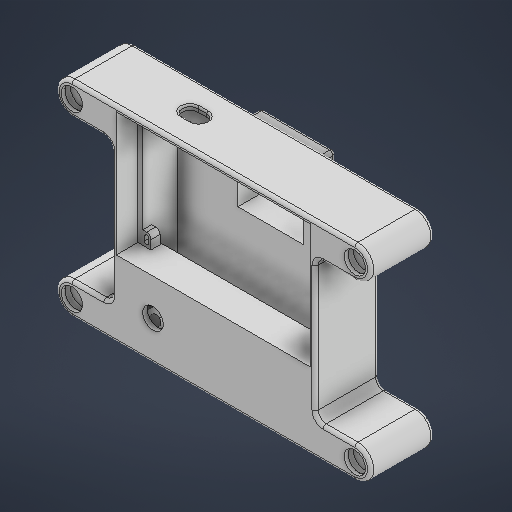
# Autodesk Inventor part: door-opener-v2-enclosure
Saved by Autodesk Inventor 2026.2 (Build 302298010, 298A)
## iProperties
Created: 2025-11-21
Part Number: door-opener-v2-enclosure
Material: Generic
Document SubType Name: Modeling
Designer: ericswpark
Density: 1 g/cm^3
Appearance: Default
Author: ericswpark
Autodesk Inventor part; units mm, degrees
ref_plane "YZ Plane" through (0, 0, 0) normal (1, 0, 0) x (0, 1, 0)
ref_plane "XZ Plane" through (0, 0, 0) normal (0, 1, 0) x (-1, 0, 0)
ref_plane "XY Plane" through (0, 0, 0) normal (0, 0, 1) x (1, 0, 0)
sketch "Sketch1" plane through (0, 0, 0) normal (0, 0, 1) x (1, 0, 0)
  line L0 (0, 0) -> (128.3, 0)
  line L1 (128.3, 0) -> (128.3, 129.1)
  line L2 (128.3, 129.1) -> (0, 129.1)
  line L3 (0, 129.1) -> (0, 0)
  circle A0 centre (153.3, 119.1) radius 10
  line L4 (128.3, 129.1) -> (153.3, 129.1)
  line L5 (153.3, 129.1) -> (153.3, 109.1)
  line L6 (153.3, 109.1) -> (128.3, 109.1)
  line L7 (128.3, 109.1) -> (128.3, 129.1)
  circle A1 centre (153.3, 119.1) radius 7
  circle A2 centre (-25, 119.1) radius 7
  circle A3 centre (-25, 119.1) radius 10
  line L8 (-25, 109.1) -> (0, 109.1)
  line L9 (0, 109.1) -> (0, 129.1)
  line L10 (0, 129.1) -> (-25, 129.1)
  line L11 (-25, 129.1) -> (-25, 109.1)
  circle A4 centre (153.3, 10) radius 7
  circle A5 centre (153.3, 10) radius 10
  line L12 (153.3, 20) -> (128.3, 20)
  line L13 (128.3, 20) -> (128.3, 0)
  line L14 (128.3, 0) -> (153.3, 0)
  line L15 (153.3, 0) -> (153.3, 20)
  line L16 (0, 20) -> (-25, 20)
  line L17 (-25, 20) -> (-25, 0)
  line L18 (-25, 0) -> (0, 0)
  line L19 (0, 0) -> (0, 20)
  circle A6 centre (-25, 10) radius 7
  circle A7 centre (-25, 10) radius 10
  point P0 (153.3, 0)
  point P1 (0, 20)
  point P2 (-25, 129.1)
  point P3 (-25, 109.1)
  point P4 (0, 109.1)
  point P5 (128.3, 109.1)
  point P6 (153.3, 109.1)
  point P7 (153.3, 129.1)
  dimension "d0" = 128.3
  dimension "d1" = 129.1
  dimension "d87" = 25
  dimension "d88" = 20
  dimension "d89" = 14
  dimension "d90" = 14
  dimension "d91" = 20
  dimension "d92" = 25
  dimension "d93" = 14
  dimension "d94" = 20
  dimension "d95" = 25
  dimension "d96" = 14
  dimension "d97" = 20
  dimension "d98" = 25
  constraints: 40 end point, 10 parallel, 8 centre point, 8 tangent, 6 midpoint, 5 horizontal, 5 perpendicular, 4 coincident, 3 point on line
  measures "d0" distance between parallel lines of L1 L3
  measures "d1" distance between parallel lines of L0 L2
  measures "d87" distance from line of L1 point (153.3, 119.1)
  measures "d88" diameter of A0
  measures "d89" diameter of A1
  measures "d90" diameter of A2
  measures "d91" diameter of A3
  measures "d92" distance from line of L3 point (-25, 119.1)
  measures "d93" diameter of A6
  measures "d94" diameter of A7
  measures "d95" distance from line of L3 A6.centre
  measures "d96" diameter of A4
  measures "d97" diameter of A5
  measures "d98" distance from line of L1 A4.centre
extrude "Initial extrusion" add sketch "Sketch1" along normal blind 40
sketch "Sketch2" plane through (0, 0, 0) normal (0, 0, -1) x (-1, 0, 0)
  line L0 (-6, 0) -> (-122.3, 0)
  line L1 (-122.3, 0) -> (-122.3, 123.1)
  line L2 (-122.3, 123.1) -> (-6, 123.1)
  line L3 (-6, 123.1) -> (-6, 0)
  line L4 (0, 109.1) -> (0, 0) projected
  line L5 (-128.3, 20) -> (-128.3, 109.1) projected
  line L6 (-153.3, 129.1) -> (25, 129.1) projected
  line L7 (25, 0) -> (-153.3, 0) projected
  dimension "d4" = 6
  dimension "d5" = 6
  dimension "d180" = 6
  constraints: 8 end point, 2 parallel, 1 collinear, 1 horizontal, 1 perpendicular
  measures "d4" distance between parallel lines of L4 L3
  measures "d5" distance between parallel lines of L1 L5
  measures "d180" distance between parallel lines of L2 L6
extrude "Top cutout" cut sketch "Sketch2" against normal blind 3
sketch "Sketch3" plane through (0, 0, 40) normal (0, -1, 0) x (1, 0, 0)
  line L0 (125.3, -37) -> (3, -37)
  line L1 (3, -37) -> (3, -35.5)
  line L2 (3, -35.5) -> (125.3, -35.5)
  line L3 (125.3, -35.5) -> (125.3, -37)
  line L4 (6, -37) -> (122.3, -37) projected
  line L5 (122.3, -37) -> (122.3, -40) projected
  line L6 (6, -40) -> (6, -37) projected
  dimension "d11" = 1.5
  dimension "d181" = 3
  dimension "d182" = 3
  constraints: 8 end point, 2 parallel, 1 collinear, 1 horizontal, 1 perpendicular
  measures "d11" distance between parallel lines of L0 L2
  measures "d181" distance between parallel lines of L5 L3
  measures "d182" distance between parallel lines of L1 L6
extrude "BP slide section" cut sketch "Sketch3" against normal blind 126.6
sketch "Sketch4" plane through (125.3, 0, 4.5) normal (0, 0, -1) x (-1, 0, 0)
  line L0 (119.3, 3) -> (3, 3)
  line L1 (3, 3) -> (3, 126.1)
  line L2 (3, 126.1) -> (119.3, 126.1)
  line L3 (119.3, 126.1) -> (119.3, 3)
  line L4 (0, 0) -> (0, 126.6) projected
  line L5 (122.3, 0) -> (122.3, 126.6) projected
  line L6 (122.3, 0) -> (0, 0) projected
  line L7 (-28, 129.1) -> (150.3, 129.1) projected
  point P0 (125.3, 0)
  point P1 (0, 123.1)
  dimension "d15" = 3
  dimension "d16" = 3
  dimension "d183" = 3
  dimension "d184" = 3
  constraints: 8 end point, 2 parallel, 1 horizontal, 1 perpendicular
  measures "d15" distance between parallel lines of L1 L4
  measures "d16" distance between parallel lines of L5 L3
  measures "d183" distance between parallel lines of L6 L0
  measures "d184" distance between parallel lines of L2 L7
extrude "Inner cavity" cut sketch "Sketch4" against normal blind 32.5
sketch "Sketch6" plane through (125.3, 0, 37) normal (0, 0, -1) x (-1, 0, 0)
  circle A0 centre (5.5, 121) radius 2.75
  circle A1 centre (116.8, 121) radius 2.75
  arc A2 (3, 54.7456) -> (3, 52.4544) centre (5.5, 53.6) ccw construction
  line L0 (3, 126.1) -> (119.3, 126.1) projected
  line L1 (3, 3) -> (3, 126.1) projected
  line L2 (119.3, 126.1) -> (119.3, 3) projected
  line L3 (3, 0) -> (3, 126.1) projected
  line L4 (3, 50.85) -> (3, 56.35)
  line L5 (3, 56.35) -> (5.5, 56.35)
  line L6 (5.5, 56.35) -> (5.5, 50.85) construction
  line L7 (3, 126.1) -> (8.25, 126.1)
  line L8 (8.25, 126.1) -> (8.25, 118.25)
  line L9 (8.25, 118.25) -> (3, 118.25)
  line L10 (3, 118.25) -> (3, 126.1)
  line L11 (119.3, 126.1) -> (114.05, 126.1)
  line L12 (114.05, 126.1) -> (114.05, 118.25)
  line L13 (114.05, 118.25) -> (119.3, 118.25)
  line L14 (119.3, 118.25) -> (119.3, 126.1)
  arc A3 (6.85, 53.6) -> (4.15, 53.6) centre (5.5, 53.6) ccw
  circle A4 centre (116.8, 121) radius 1.35
  circle A5 centre (5.5, 121) radius 1.35
  line L15 (3, 56.35) -> (8.25, 56.35) construction
  line L16 (8.25, 56.35) -> (8.25, 53.6) construction
  line L17 (8.25, 48) -> (3, 48)
  line L18 (3, 48) -> (3, 56.35)
  line L19 (8.25, 53.6) -> (8.25, 48)
  arc A6 (5.5, 56.35) -> (3, 54.7456) centre (5.5, 53.6) ccw construction
  arc A7 (3, 52.4544) -> (8.25, 53.6) centre (5.5, 53.6) ccw construction
  arc A8 (8.25, 53.6) -> (5.5, 56.35) centre (5.5, 53.6) ccw
  line L20 (4.15, 53.6) -> (6.85, 53.6) construction
  line L21 (6.85, 53.6) -> (6.85, 50.85)
  line L22 (5.5, 50.85) -> (4.15, 50.85) construction
  line L23 (4.15, 50.85) -> (4.15, 53.6)
  line L24 (4.15, 50.85) -> (3, 50.85) construction
  arc A9 (4.15, 50.85) -> (6.85, 50.85) centre (5.5, 50.85) ccw
  line L25 (116.8, 121) -> (5.5, 121) construction
  line L26 (61.15, 121) -> (61.15, 42.4019) construction
  arc A10 (119.3, 52.4544) -> (119.3, 54.7456) centre (116.8, 53.6) ccw construction
  line L27 (119.3, 3) -> (119.3, 126.1)
  line L28 (119.3, 50.85) -> (119.3, 56.35)
  line L29 (119.3, 56.35) -> (116.8, 56.35)
  line L30 (116.8, 56.35) -> (116.8, 50.85) construction
  arc A11 (118.15, 53.6) -> (115.45, 53.6) centre (116.8, 53.6) ccw
  line L31 (119.3, 56.35) -> (114.05, 56.35) construction
  line L32 (114.05, 56.35) -> (114.05, 53.6) construction
  line L33 (114.05, 48) -> (119.3, 48)
  line L34 (119.3, 48) -> (119.3, 56.35)
  line L35 (114.05, 53.6) -> (114.05, 48)
  arc A12 (119.3, 54.7456) -> (116.8, 56.35) centre (116.8, 53.6) ccw construction
  arc A13 (114.05, 53.6) -> (119.3, 52.4544) centre (116.8, 53.6) ccw construction
  arc A14 (116.8, 56.35) -> (114.05, 53.6) centre (116.8, 53.6) ccw
  line L36 (118.15, 53.6) -> (115.45, 53.6) construction
  line L37 (115.45, 53.6) -> (115.45, 50.85)
  line L38 (116.8, 50.85) -> (118.15, 50.85) construction
  line L39 (118.15, 50.85) -> (118.15, 53.6)
  line L40 (118.15, 50.85) -> (119.3, 50.85) construction
  arc A15 (115.45, 50.85) -> (118.15, 50.85) centre (116.8, 50.85) ccw
  point P0 (125.3, 0)
  point P1 (1, 0)
  point P2 (5.5, 56.35)
  point P3 (3, 56.35)
  point P4 (114.05, 121)
  point P5 (116.8, 118.25)
  point P6 (5.5, 118.25)
  point P7 (8.25, 121)
  point P8 (3, 118.25)
  point P9 (3, 48)
  dimension "d26" = 5.1
  dimension "d27" = 2.5
  dimension "d28" = 5.1
  dimension "d29" = 2.5
  dimension "d34" = 5.5
  dimension "d35" = 5.5
  dimension "d46" = 2.7
  dimension "d48" = 2.7
  dimension "d49" = 2.7
  dimension "d178" = 2.5
  dimension "d179" = 5.5
  dimension "d190" = 67.4
  dimension "d211" = 2.85
  dimension "d212" = 78.5981
  constraints: 74 end point, 26 point on circle, 18 symmetric about line, 18 tangent, 16 centre point, 11 parallel, 6 coincident, 6 midpoint, 6 perpendicular, 5 horizontal, 2 point on line, 1 collinear, 1 vertical, 8 other
  measures "d26" distance from line of L0 A0.centre
  measures "d27" distance from line of L1 A0.centre
  measures "d28" distance from line of L0 A1.centre
  measures "d29" distance from line of L2 A1.centre
  measures "d34" diameter of A0
  measures "d35" diameter of A1
  measures "d46" diameter of A3
  measures "d48" diameter of A4
  measures "d49" diameter of A5
  measures "d178" distance from line of L1 A3.centre
  measures "d179" diameter of A2
  measures "d190" distance of point (5.5, 53.6) A0.centre
  measures "d211" distance between parallel lines of L17 L24
  measures "d212" distance of L26.start L26.end
extrude "Display mount holes" add sketch "Sketch6" along normal blind 16.3 contours A0 L1 | A0 L1 L0 L8 | L9 L1 A0 | L2 A1 | A1 L12 L0 L2 | L2 L13 A1 | L1 L5 A8 L19 L17 | L2 L33 L35 A14 L29 picked at (3.3833, 121) picked at (118.9167, 121)
sketch "Sketch7" plane through (0, 0, 40) normal (0, 0, 1) x (1, 0, 0)
  line L0 (3, 126.1) -> (125.3, 126.1)
  line L1 (125.3, 126.1) -> (125.3, 48)
  line L2 (125.3, 48) -> (3, 48)
  line L3 (3, 48) -> (3, 126.1)
  line L4 (0, 109.1) -> (0, 0) projected
  line L5 (128.3, 20) -> (128.3, 109.1) projected
  line L6 (153.3, 129.1) -> (-25, 129.1) projected
  point P0 (124.3, 0)
  dimension "d40" = 3
  dimension "d42" = 3
  dimension "d43" = 78.1
  dimension "d185" = 3
  constraints: 8 end point, 2 parallel, 1 horizontal, 1 perpendicular, 1 other
  measures "d40" distance between parallel lines of L4 L3
  measures "d43" distance between parallel lines of L0 L2
  measures "d185" distance between parallel lines of L0 L6
extrude "Display cutout" cut sketch "Sketch7" against normal blind 13.6
sketch "Sketch9" plane through (125.3, 0, 37) normal (0, 0, -1) x (-1, 0, 0)
  line L0 (3, 3) -> (3, 48) projected
  line L1 (119.3, 48) -> (119.3, 3) projected
  line L2 (3, 48) -> (119.3, 48)
  line L3 (119.3, 48) -> (119.3, 46)
  line L4 (119.3, 46) -> (3, 46)
  line L5 (3, 46) -> (3, 48)
  point P0 (125.3, 0)
  point P1 (119.3, 48)
  point P2 (3, 46)
  dimension "d50" = 2
  constraints: 8 end point, 2 parallel, 1 horizontal, 1 perpendicular, 1 point on line
  measures "d50" distance between parallel lines of L2 L4
extrude "Separator" add sketch "Sketch9" along normal blind 17.5
sketch "Sketch10" plane through (125.3, 0, 37) normal (0, 0, -1) x (-1, 0, 0)
  circle A0 centre (11, 38) radius 2.25
  circle A1 centre (39, 12) radius 2.25
  circle A2 centre (39, 12) radius 3.25
  circle A3 centre (11, 38) radius 3.25
  line L0 (119.3, 46) -> (3, 46) projected
  line L1 (3, 3) -> (3, 46) projected
  point P0 (125.3, 0)
  dimension "d53" = 4.5
  dimension "d54" = 6.5
  dimension "d55" = 8
  dimension "d56" = 8
  dimension "d57" = 4.5
  dimension "d58" = 6.5
  dimension "d59" = 28
  dimension "d60" = 26
  constraints: 4 centre point, 2 coincident
  measures "d53" diameter of A0
  measures "d54" diameter of A3
  measures "d55" distance from line of A0.centre L0
  measures "d56" distance from line of L1 A0.centre
  measures "d57" diameter of A1
  measures "d58" diameter of A2
  measures "d59" horizontal distance of A0.centre A1.centre
  measures "d60" vertical distance of A0.centre A1.centre
extrude "NFC reader mount holes" add sketch "Sketch10" along normal blind 3
sketch "Camera mount hole sketch" plane through (125.3, 0, 37) normal (0, 0, -1) x (-1, 0, 0)
  circle A0 centre (109.3, 13) radius 1.6
  circle A1 centre (109.3, 13) radius 3.1
  circle A2 centre (89.1, 13) radius 1.6
  circle A3 centre (89.1, 13) radius 3.1
  circle A4 centre (109.3, 25) radius 1.6
  circle A5 centre (109.3, 25) radius 3.1
  circle A6 centre (89.1, 25) radius 1.6
  circle A7 centre (89.1, 25) radius 3.1
  line L0 (119.3, 46) -> (119.3, 3) projected
  line L1 (119.3, 3) -> (3, 3) projected
  circle A8 centre (99.2, 25) radius 6.5
  line L2 (89.1, 25) -> (109.3, 25)
  point P0 (125.3, 0)
  dimension "d63" = 3.2
  dimension "d64" = 6.2
  dimension "d65" = 3.2
  dimension "d66" = 6.2
  dimension "d67" = 6.2
  dimension "d68" = 6.2
  dimension "d69" = 3.2
  dimension "d70" = 3.2
  dimension "d72" = 20.2
  dimension "d73" = 12
  dimension "d74" = 20.2
  dimension "d75" = 12
  dimension "d76" = 0
  dimension "d77" = 0
  dimension "d78" = 10
  dimension "d79" = 10
  dimension "d82" = 10.1
  dimension "d83" = 0
  dimension "d84" = 13
  constraints: 9 centre point, 4 coincident, 2 end point
  measures "d63" diameter of A6
  measures "d64" diameter of A7
  measures "d65" diameter of A4
  measures "d66" diameter of A5
  measures "d67" diameter of A3
  measures "d68" diameter of A1
  measures "d69" diameter of A2
  measures "d70" diameter of A0
  measures "d72" distance of A4.centre A6.centre
  measures "d73" distance of A0.centre A4.centre
  measures "d74" distance of A2.centre A0.centre
  measures "d75" distance of A6.centre A2.centre
  measures "d76" horizontal distance of A2.centre A6.centre
  measures "d77" vertical distance of A6.centre A4.centre
  measures "d78" distance from line of L0 A1.centre
  measures "d79" distance from line of L1 A0.centre
  measures "d82" distance of A8.centre A6.centre
  measures "d83" vertical distance of A6.centre A8.centre
  measures "d84" diameter of A8
extrude "Camera mount holes" add sketch "Camera mount hole sketch" along normal blind 9 contours A1 | A3 | A5 | A7
extrude "Camera mount hole inner offset extrude" add sketch "Camera mount hole sketch" along normal blind 6.5 contours A0 | A2 | A4 | A6
extrude "Camera cutout" cut sketch "Camera mount hole sketch" against normal blind 3 contours L2 A8 | A8 L2
sketch "Sketch13" plane through (0, 0, 40) normal (0, 0, 1) x (1, 0, 0)
  circle A0 centre (-25, 119.1) radius 6.75
  circle A1 centre (-25, 10) radius 6.75
  circle A2 centre (153.3, 10) radius 6.75
  circle A3 centre (153.3, 119.1) radius 6.75
  line L0 (125.3, 126.1) -> (125.3, 48) projected
  line L1 (128.3, 109.1) -> (153.3, 109.1) projected
  line L2 (3, 48) -> (3, 126.1) projected
  line L3 (-25, 109.1) -> (0, 109.1) projected
  line L4 (153.3, 20) -> (128.3, 20) projected
  line L5 (128.3, 20) -> (128.3, 109.1) projected
  line L6 (0, 109.1) -> (0, 20) projected
  line L7 (0, 20) -> (-25, 20) projected
  point P0 (0, 0)
  dimension "d126" = 13.5
  dimension "d127" = 10
  dimension "d128" = 13.5
  dimension "d130" = 10
  dimension "d131" = 10
  dimension "d132" = 13.5
  dimension "d133" = 25
  dimension "d134" = 25
  dimension "d135" = 25
  dimension "d136" = 25
  dimension "d137" = 13.5
  dimension "d138" = 10
  constraints: 4 centre point
  measures "d126" diameter of A3
  measures "d127" distance from line of L1 A3.centre
  measures "d128" diameter of A0
  measures "d130" distance from line of L3 A0.centre
  measures "d131" distance from line of L4 A2.centre
  measures "d132" diameter of A2
  measures "d133" distance from line of L5 A2.centre
  measures "d134" distance from line of L5 A3.centre
  measures "d135" distance from line of L6 A0.centre
  measures "d136" distance from line of L6 A1.centre
  measures "d137" diameter of A1
  measures "d138" distance from line of L7 A1.centre
extrude "Suction cup holes" cut sketch "Sketch13" against normal blind 6.2
ref_plane "Suction cup cutout reference plane" through (0, 0, 37.6) normal (0, 0, 1) x (1, 0, 0)
sketch "Sketch14" plane through (0, 0, 37.6) normal (0, 0, 1) x (1, 0, 0)
  circle A0 centre (-25, 119.1) radius 6.75 projected
  circle A1 centre (-25, 119.1) radius 7.25
  circle A2 centre (153.3, 119.1) radius 6.75 projected
  circle A3 centre (153.3, 119.1) radius 7.25
  circle A4 centre (153.3, 10) radius 6.75 projected
  circle A5 centre (153.3, 10) radius 7.25
  circle A6 centre (-25, 10) radius 6.75 projected
  circle A7 centre (-25, 10) radius 7.25
  point P0 (0, 0)
  dimension "d142" = 14.5
  dimension "d143" = 14.5
  dimension "d144" = 14.5
  dimension "d145" = 14.5
  constraints: 4 centre point, 4 coincident
  measures "d142" diameter of A1
  measures "d143" diameter of A7
  measures "d144" diameter of A5
  measures "d145" diameter of A3
extrude "Suction cup inner nub cut" cut sketch "Sketch14" against normal blind 3.8
sketch "Sketch16" plane through (0, 126.6, 40) normal (0, -1, 0) x (1, 0, 0)
  line L0 (124.3, -36) -> (124.3, -37.0114)
  line L1 (4, -36.75) -> (4, -35.4223)
  line L2 (124.3, -36) -> (4, -36)
  line L3 (4, -36) -> (4, -36.75)
  line L4 (4, -36.75) -> (124.3, -36.75)
  line L5 (124.3, -36.75) -> (124.3, -36)
  line L6 (125.3, -35.5) -> (125.3, -37) projected
  line L7 (3, -35.5) -> (125.3, -35.5) projected
  line L8 (3, -37) -> (3, -35.5) projected
  line L9 (125.3, -37) -> (3, -37) projected
  point P0 (0, -40)
  point P1 (4, -36)
  point P2 (122.3, -35.5)
  dimension "d196" = 1
  dimension "d197" = 0.5
  dimension "d198" = 1
  dimension "d199" = 0.25
  constraints: 12 end point, 2 parallel, 1 perpendicular
  measures "d196" distance between parallel lines of L0 L6
  measures "d197" distance between parallel lines of L7 L2
  measures "d198" distance between parallel lines of L8 L1
  measures "d199" distance between parallel lines of L9 L4
extrude "BackPlate inner" add sketch "Sketch16" along normal blind 126.1 separate body contours L0 L4 L1 L2
sketch "Sketch17" plane through (124.3, 126.6, 3.25) normal (0, 0, -1) x (-1, 0, 0)
  line L0 (2.5, -126.1) -> (2.5, -4)
  line L1 (2.5, -4) -> (117.8, -4)
  line L2 (117.8, -4) -> (117.8, -126.1)
  line L3 (0, 0) -> (0, -126.1) projected
  line L4 (121.3, -126.6) -> (121.3, 0) projected
  line L5 (118.3, -3.5) -> (118.3, -126.6) projected
  line L6 (2, -126.6) -> (2, -3.5) projected
  line L7 (2, -3.5) -> (118.3, -3.5) projected
  line L8 (2.5, -126.1) -> (117.8, -126.1)
  line L9 (120.3, -126.1) -> (0, -126.1) projected
  dimension "d201" = 0.5
  dimension "d202" = 0.5
  dimension "d203" = 0.5
  constraints: 8 end point, 2 parallel, 1 horizontal, 1 perpendicular, 1 other
  measures "d201" distance between parallel lines of L2 L5
  measures "d202" distance between parallel lines of L0 L6
  measures "d203" distance between parallel lines of L1 L7
extrude "BackPlate outer" add sketch "Sketch17" along normal blind 3 contours L0 L1 L2 L8 bodies 2
sketch "Sketch19" plane through (6, 126.1, 4.5) normal (0, -1, 0) x (1, 0, 0)
  line L0 (23, 15) -> (28.5, 15) construction
  line L1 (23, 10) -> (28.5, 10)
  line L2 (28.5, 20) -> (23, 20)
  arc A0 (23, 20) -> (23, 10) centre (23, 15) ccw
  arc A1 (28.5, 10) -> (28.5, 20) centre (28.5, 15) ccw
  line L3 (-3, 35.5) -> (119.3, 35.5) projected
  line L4 (-3, 35.5) -> (-3, 21.9) projected
  point P0 (-6, -4.5)
  point P1 (25.75, 15)
  point P2 (18, 15)
  point P3 (33.5, 15)
  dimension "d158" = 10
  dimension "d159" = 15.5
  dimension "d204" = 15.5
  dimension "d205" = 21
  constraints: 8 end point, 6 point on circle, 4 tangent, 2 centre point, 1 horizontal, 1 midpoint, 1 parallel
  measures "d158" distance between parallel lines of L1 L2
  measures "d159" distance of point (33.5, 15) point (18, 15)
  measures "d204" distance between parallel lines of L2 L3
  measures "d205" distance from line of point (18, 15) L4
extrude "USB-C cutout" cut sketch "Sketch19" against normal blind 15 bodies 1
sketch "Sketch20" plane through (125.3, 0, 37) normal (0, 0, -1) x (-1, 0, 0)
  circle A0 centre (63.15, 8.25) radius 2.25
  circle A1 centre (63.15, 8.25) radius 3.25
  line L0 (119.3, 3) -> (3, 3) projected
  line L1 (3, 3) -> (3, 46) projected
  line L2 (119.3, 46) -> (119.3, 3) projected
  line L3 (66.4, 3) -> (59.9, 3)
  line L4 (59.9, 3) -> (59.9, 8.25)
  line L5 (59.9, 8.25) -> (66.4, 8.25)
  line L6 (66.4, 8.25) -> (66.4, 3)
  point P0 (125.3, 0)
  point P1 (66.4, 8.25)
  point P2 (59.9, 3)
  dimension "d162" = 4.5
  dimension "d163" = 6.5
  dimension "d165" = 2
  dimension "d166" = 60.15
  dimension "d167" = 56.15
  constraints: 8 end point, 2 centre point, 2 parallel, 2 tangent, 1 coincident, 1 horizontal, 1 midpoint, 1 perpendicular, 1 point on line
  measures "d162" diameter of A0
  measures "d163" diameter of A1
  measures "d165" distance edge to line of A1 L0
  measures "d166" distance from line of L1 A0.centre
  measures "d167" distance from line of L2 A0.centre
extrude "Enclosure BP screw mount" add sketch "Sketch20" along normal blind 32 contours L5 A1 A0 | A0 L5 A1 | L6 L0 L4 A1 bodies 1
sketch "Sketch22" plane through (62.15, 8.25, 37) normal (0, 0, -1) x (-1, 0, 0)
  circle A0 centre (0, 0) radius 2.25 projected
  circle A1 centre (0, 0) radius 2.25
  point P0 (62.15, -8.25)
  constraints: 1 centre point, 1 coincident, 1 concentric
extrude "Enclosure BP screw mount hole" add sketch "Sketch22" along normal blind 29 bodies 1
sketch "Sketch23" plane through (124.3, 126.6, 0.25) normal (0, 0, -1) x (-1, 0, 0)
  circle A0 centre (62.15, -118.35) radius 2.25
  line L0 (2.5, -126.1) -> (117.8, -126.1) projected
  line L1 (118.3, -123.6) -> (2, -123.6) projected
  line L2 (2, -126.6) -> (2, -3.5) projected
  point P0 (124.3, -126.6)
  point P1 (1, -124.1)
  point P2 (117.8, -126.1)
  point P3 (2, -3.5)
  dimension "d172" = 4.5
  dimension "d174" = 3
  dimension "d175" = 60.15
  constraints: 1 centre point, 2 other
  measures "d172" diameter of A0
  measures "d174" distance edge to line of A0 L1
extrude "BackPlate screw hole" cut sketch "Sketch23" against normal blind 4.5 bodies 2
fillet "Suction cup arm fillets" radius 5 4 edges at (128.3, 109.1, 20) (128.3, 20, 20) (0, 109.1, 20) (0, 20, 20)
fillet "Front-back fillets" radius 2 34 edges at (137.8, 0, 0) (163.3, 10, 0) (143.3, 20, 0) (129.7645, 21.4645, 0) (128.3, 64.55, 0) (129.7645, 107.6355, 0) (143.3, 109.1, 0) (163.3, 119.1, 0) (64.15, 129.1, 0) (-35, 119.1, 0) (-15, 109.1, 0) (-1.4645, 107.6355, 0) (0, 64.55, 0) (-1.4645, 21.4645, 0) (-15, 20, 0) (-35, 10, 0) (-9.5, 0, 0) (64.15, 0, 40) (163.3, 10, 40) (143.3, 20, 40) (129.7645, 21.4645, 40) (128.3, 64.55, 40) (129.7645, 107.6355, 40) (143.3, 109.1, 40) (163.3, 119.1, 40) (64.15, 129.1, 40) (-35, 119.1, 40) (-15, 109.1, 40) (-1.4645, 107.6355, 40) (0, 64.55, 40) (-1.4645, 21.4645, 40) (-15, 20, 40) (-35, 10, 40) (64.15, 0.5, 0.25)
fillet "USB-C port fillet" radius 1 4 edges at (31.75, 129.1, 14.5) (39.5, 129.1, 19.5) (31.75, 129.1, 24.5) (24, 129.1, 19.5)
sketch "Sketch24" plane through (124.3, 126.6, 0.25) normal (0, 0, -1) x (-1, 0, 0)
  line L0 (2.5, -9) -> (117.8, -9) construction
  line L1 (117.8, -124.1) -> (117.8, -4) construction
  line L2 (2.5, -4) -> (2.5, -124.1) construction
  line L3 (117.8, -4) -> (2.5, -4) construction
  line L4 (39.65, -9) -> (80.65, -9)
  line L5 (80.65, -9) -> (80.65, -50)
  line L6 (80.65, -50) -> (39.65, -50)
  line L7 (39.65, -50) -> (39.65, -9)
  point P0 (124.3, -126.6)
  point P1 (60.15, -9)
  dimension "d213" = 5
  dimension "d214" = 41
  dimension "d215" = 41
  constraints: 10 end point, 3 point on line, 2 midpoint, 2 parallel, 2 perpendicular, 1 horizontal
  measures "d213" distance between parallel lines of L0 L3
  measures "d214" distance of L5.end L6.end
  measures "d215" distance of L4.end L5.end
extrude "Fan Hole" cut sketch "Sketch24" against normal blind 10 bodies 2
sketch "Sketch25" plane through (124.3, 126.6, 0.25) normal (0, 0, -1) x (-1, 0, 0)
  line L0 (36.65, -6) -> (83.65, -6)
  line L1 (83.65, -6) -> (83.65, -53)
  line L2 (83.65, -53) -> (36.65, -53)
  line L3 (36.65, -53) -> (36.65, -6)
  line L4 (80.65, -9) -> (80.65, -50) projected
  line L5 (39.65, -9) -> (80.65, -9) projected
  line L6 (39.65, -50) -> (39.65, -9) projected
  line L7 (80.65, -50) -> (39.65, -50) projected
  point P0 (124.3, -126.6)
  dimension "d218" = 3
  dimension "d219" = 3
  dimension "d220" = 3
  dimension "d221" = 3
  constraints: 8 end point, 2 parallel, 1 horizontal, 1 perpendicular
  measures "d218" distance between parallel lines of L1 L4
  measures "d219" distance between parallel lines of L5 L0
  measures "d220" distance between parallel lines of L3 L6
  measures "d221" distance between parallel lines of L2 L7
extrude "Fan Holder Walls" add sketch "Sketch25" along normal blind 11 bodies 2
sketch "Sketch26" plane through (124.3, 126.6, -10.75) normal (0, 0, -1) x (-1, 0, 0)
  line L0 (36.65, -6) -> (36.65, -53) projected
  line L1 (83.65, -6) -> (36.65, -6) projected
  line L2 (83.65, -53) -> (83.65, -6) projected
  line L3 (36.65, -53) -> (83.65, -53) projected
  point P0 (124.3, -126.6)
extrude "Fan Back Plate" add sketch "Sketch26" along normal blind 3 bodies 2
sketch "Sketch27" plane through (124.3, 126.6, -13.75) normal (0, 0, -1) x (-1, 0, 0)
  line L0 (39.65, -50) -> (39.65, -9) projected
  line L1 (39.65, -9) -> (80.65, -9) projected
  line L2 (80.65, -9) -> (80.65, -50) projected
  line L3 (80.65, -50) -> (39.65, -50) projected
  line L4 (39.65, -9) -> (39.65, -50) construction
  line L5 (39.65, -29.5) -> (80.65, -29.5) construction
  line L6 (60.15, -9) -> (60.15, -50) construction
  circle A0 centre (60.15, -29.5) radius 1.5
  circle A1 centre (60.15, -33.5) radius 1.5
  circle A2 centre (60.15, -25.5) radius 1.5
  circle A3 centre (60.15, -37.5) radius 1.5
  circle A4 centre (60.15, -21.5) radius 1.5
  circle A5 centre (60.15, -41.5) radius 1.5
  circle A6 centre (60.15, -17.5) radius 1.5
  circle A7 centre (60.15, -45.5) radius 1.5
  circle A8 centre (60.15, -13.5) radius 1.5
  circle A9 centre (64.15, -29.5) radius 1.5
  circle A10 centre (64.15, -33.5) radius 1.5
  circle A11 centre (64.15, -25.5) radius 1.5
  circle A12 centre (64.15, -37.5) radius 1.5
  circle A13 centre (64.15, -21.5) radius 1.5
  circle A14 centre (64.15, -41.5) radius 1.5
  circle A15 centre (64.15, -17.5) radius 1.5
  circle A16 centre (64.15, -45.5) radius 1.5
  circle A17 centre (64.15, -13.5) radius 1.5
  circle A18 centre (56.15, -29.5) radius 1.5
  circle A19 centre (56.15, -33.5) radius 1.5
  circle A20 centre (56.15, -25.5) radius 1.5
  circle A21 centre (56.15, -37.5) radius 1.5
  circle A22 centre (56.15, -21.5) radius 1.5
  circle A23 centre (56.15, -41.5) radius 1.5
  circle A24 centre (56.15, -17.5) radius 1.5
  circle A25 centre (56.15, -45.5) radius 1.5
  circle A26 centre (56.15, -13.5) radius 1.5
  circle A27 centre (68.15, -29.5) radius 1.5
  circle A28 centre (68.15, -33.5) radius 1.5
  circle A29 centre (68.15, -25.5) radius 1.5
  circle A30 centre (68.15, -37.5) radius 1.5
  circle A31 centre (68.15, -21.5) radius 1.5
  circle A32 centre (68.15, -41.5) radius 1.5
  circle A33 centre (68.15, -17.5) radius 1.5
  circle A34 centre (68.15, -45.5) radius 1.5
  circle A35 centre (68.15, -13.5) radius 1.5
  circle A36 centre (52.15, -29.5) radius 1.5
  circle A37 centre (52.15, -33.5) radius 1.5
  circle A38 centre (52.15, -25.5) radius 1.5
  circle A39 centre (52.15, -37.5) radius 1.5
  circle A40 centre (52.15, -21.5) radius 1.5
  circle A41 centre (52.15, -41.5) radius 1.5
  circle A42 centre (52.15, -17.5) radius 1.5
  circle A43 centre (52.15, -45.5) radius 1.5
  circle A44 centre (52.15, -13.5) radius 1.5
  circle A45 centre (72.15, -29.5) radius 1.5
  circle A46 centre (72.15, -33.5) radius 1.5
  circle A47 centre (72.15, -25.5) radius 1.5
  circle A48 centre (72.15, -37.5) radius 1.5
  circle A49 centre (72.15, -21.5) radius 1.5
  circle A50 centre (72.15, -41.5) radius 1.5
  circle A51 centre (72.15, -17.5) radius 1.5
  circle A52 centre (72.15, -45.5) radius 1.5
  circle A53 centre (72.15, -13.5) radius 1.5
  circle A54 centre (48.15, -29.5) radius 1.5
  circle A55 centre (48.15, -33.5) radius 1.5
  circle A56 centre (48.15, -25.5) radius 1.5
  circle A57 centre (48.15, -37.5) radius 1.5
  circle A58 centre (48.15, -21.5) radius 1.5
  circle A59 centre (48.15, -41.5) radius 1.5
  circle A60 centre (48.15, -17.5) radius 1.5
  circle A61 centre (48.15, -45.5) radius 1.5
  circle A62 centre (48.15, -13.5) radius 1.5
  circle A63 centre (76.15, -29.5) radius 1.5
  circle A64 centre (76.15, -33.5) radius 1.5
  circle A65 centre (76.15, -25.5) radius 1.5
  circle A66 centre (76.15, -37.5) radius 1.5
  circle A67 centre (76.15, -21.5) radius 1.5
  circle A68 centre (76.15, -41.5) radius 1.5
  circle A69 centre (76.15, -17.5) radius 1.5
  circle A70 centre (76.15, -45.5) radius 1.5
  circle A71 centre (76.15, -13.5) radius 1.5
  circle A72 centre (44.15, -29.5) radius 1.5
  circle A73 centre (44.15, -33.5) radius 1.5
  circle A74 centre (44.15, -25.5) radius 1.5
  circle A75 centre (44.15, -37.5) radius 1.5
  circle A76 centre (44.15, -21.5) radius 1.5
  circle A77 centre (44.15, -41.5) radius 1.5
  circle A78 centre (44.15, -17.5) radius 1.5
  circle A79 centre (44.15, -45.5) radius 1.5
  circle A80 centre (44.15, -13.5) radius 1.5
  point P0 (124.3, -126.6)
  dimension "d226" = 3
  dimension "d229" = 4
  dimension "d232" = 4
  constraints: 81 centre point, 5 midpoint, 4 end point, 1 coincident, 1 horizontal, 1 vertical, 160 other
  measures "d226" diameter of A0
  measures "d229" distance of A0.centre A1.centre
  measures "d232" distance of A0.centre A9.centre
hole "Fan Breathing Holes" at (64.15, 97.1, -13.75) at (80.15, 113.1, -13.75) at (76.15, 113.1, -13.75) at (80.15, 109.1, -13.75) at (72.15, 113.1, -13.75) at (76.15, 109.1, -13.75) at (72.15, 109.1, -13.75) at (68.15, 113.1, -13.75) at (64.15, 113.1, -13.75) at (60.15, 113.1, -13.75) at (56.15, 113.1, -13.75) at (52.15, 113.1, -13.75) at (48.15, 113.1, -13.75) at (48.15, 109.1, -13.75) at (52.15, 109.1, -13.75) at (56.15, 109.1, -13.75) at (60.15, 109.1, -13.75) at (64.15, 109.1, -13.75) at (68.15, 109.1, -13.75) at (68.15, 105.1, -13.75) at (72.15, 105.1, -13.75) at (76.15, 105.1, -13.75) at (80.15, 105.1, -13.75) at (80.15, 101.1, -13.75) at (76.15, 101.1, -13.75) at (72.15, 101.1, -13.75) at (68.15, 101.1, -13.75) at (64.15, 101.1, -13.75) at (60.15, 101.1, -13.75) at (64.15, 105.1, -13.75) at (60.15, 105.1, -13.75) at (56.15, 105.1, -13.75) at (56.15, 101.1, -13.75) at (52.15, 105.1, -13.75) at (52.15, 101.1, -13.75) at (48.15, 105.1, -13.75) at (48.15, 101.1, -13.75) at (48.15, 97.1, -13.75) at (52.15, 97.1, -13.75) at (56.15, 97.1, -13.75) at (60.15, 97.1, -13.75) at (68.15, 97.1, -13.75) at (72.15, 97.1, -13.75) at (76.15, 97.1, -13.75) at (80.15, 97.1, -13.75) at (80.15, 93.1, -13.75) at (76.15, 93.1, -13.75) at (72.15, 93.1, -13.75) at (68.15, 93.1, -13.75) at (64.15, 93.1, -13.75) direction (0, 0, 1) diameter 3 end through all bodies 2 and at (60.15, 93.1, -13.75) (56.15, 93.1, -13.75) (52.15, 93.1, -13.75) (48.15, 93.1, -13.75) (48.15, 89.1, -13.75) (48.15, 85.1, -13.75) (48.15, 81.1, -13.75) (52.15, 81.1, -13.75) (52.15, 85.1, -13.75) (52.15, 89.1, -13.75) (56.15, 89.1, -13.75) (56.15, 85.1, -13.75) (56.15, 81.1, -13.75) (60.15, 81.1, -13.75) (60.15, 85.1, -13.75) (60.15, 89.1, -13.75) (64.15, 89.1, -13.75) (64.15, 85.1, -13.75) (64.15, 81.1, -13.75) (68.15, 89.1, -13.75) (68.15, 85.1, -13.75) (68.15, 81.1, -13.75) (72.15, 89.1, -13.75) (72.15, 85.1, -13.75) (72.15, 81.1, -13.75) (76.15, 89.1, -13.75) (76.15, 85.1, -13.75) (76.15, 81.1, -13.75) (80.15, 89.1, -13.75) (80.15, 85.1, -13.75) (80.15, 81.1, -13.75)
fillet "Fan tumor fillets" radius 2 12 edges at (87.65, 120.6, -6.75) (87.65, 97.1, -13.75) (87.65, 73.6, -6.75) (64.15, 73.6, -13.75) (87.65, 97.1, 0.25) (64.15, 73.6, 0.25) (64.15, 120.6, 0.25) (64.15, 120.6, -13.75) (40.65, 120.6, -6.75) (40.65, 97.1, 0.25) (40.65, 97.1, -13.75) (40.65, 73.6, -6.75)
equation "\"d0\" = enclosure_total_width"
equation "\"d1\" = enclosure_total_height"
equation "\"d2\" = enclosure_thickness"
equation "\"d4\" = 2 * wall_thickness"
equation "\"d5\" = 2 * wall_thickness"
equation "\"d7\" = enclosure_back_and_plate_distance"
equation "\"d11\" = enclosure_back_plate_thickness"
equation "\"d15\" = wall_thickness"
equation "\"d16\" = wall_thickness"
equation "\"d18\" = enclosure_thickness - 2 * wall_thickness - enclosure_back_plate_thickness"
equation "\"d34\" = rpi_screen_screw_post_diameter"
equation "\"d35\" = rpi_screen_screw_post_diameter"
equation "\"d38\" = rpi_screen_screw_post_depth + rpi_screen_screw_resting_plate_thickness"
equation "\"d40\" = wall_thickness"
equation "\"d42\" = wall_thickness"
equation "\"d43\" = rpi_screen_height"
equation "\"d44\" = rpi_screen_screw_post_depth"
equation "\"d50\" = separator_wall_between_rpi_and_modules"
equation "\"d53\" = nfc_module_standoff_inner_diameter"
equation "\"d54\" = nfc_module_standoff_inner_diameter + nfc_module_standoff_thickness"
equation "\"d55\" = nfc_module_screw_hole_side_distance + tolerances"
equation "\"d56\" = nfc_module_screw_hole_side_distance + tolerances"
equation "\"d57\" = nfc_module_standoff_inner_diameter"
equation "\"d58\" = nfc_module_standoff_inner_diameter + nfc_module_standoff_thickness"
equation "\"d59\" = nfc_module_width - 2 * nfc_module_screw_hole_side_distance"
equation "\"d60\" = nfc_module_height - 2 * nfc_module_screw_hole_side_distance"
equation "\"d61\" = nfc_module_standoff_depth"
equation "\"d63\" = rpi_camera_standoff_inner_diameter"
equation "\"d64\" = rpi_camera_standoff_inner_diameter + rpi_camera_standoff_thickness"
equation "\"d65\" = rpi_camera_standoff_inner_diameter"
equation "\"d66\" = rpi_camera_standoff_inner_diameter + rpi_camera_standoff_thickness"
equation "\"d67\" = rpi_camera_standoff_inner_diameter + rpi_camera_standoff_thickness"
equation "\"d68\" = rpi_camera_standoff_inner_diameter + rpi_camera_standoff_thickness"
equation "\"d69\" = rpi_camera_standoff_inner_diameter"
equation "\"d70\" = rpi_camera_standoff_inner_diameter"
equation "\"d72\" = rpi_camera_screw_hole_horizontal_apart"
equation "\"d73\" = rpi_camera_screw_hole_vertical_apart"
equation "\"d74\" = rpi_camera_screw_hole_horizontal_apart"
equation "\"d75\" = rpi_camera_screw_hole_vertical_apart"
equation "\"d78\" = rpi_camera_bottom_right_placement"
equation "\"d79\" = rpi_camera_bottom_right_placement"
equation "\"rpi_screen_width\" = 121.3"
equation "\"rpi_screen_height\" = 78.1"
equation "\"rpi_screen_assembly_thickness\" = 32.8"
equation "\"tolerances\" = 0.5"
equation "\"wall_thickness\" = 3"
equation "\"rpi_camera_height\" = 24"
equation "\"rpi_camera_width\" = 25"
equation "\"rpi_camera_thickness\" = 12.7"
equation "\"nfc_module_height\" = 41"
equation "\"nfc_module_width\" = 43"
equation "\"nfc_module_screw_hole_side_distance\" = 7.5"
equation "\"nfc_module_screw_hole_diameter\" = 3"
equation "\"rpi_camera_screw_hole_diameter\" = 2"
equation "\"separator_wall_between_rpi_and_modules\" = 2"
equation "\"enclosure_total_height\" = 4 * tolerances + 2 * wall_thickness + rpi_screen_height + separator_wall_between_rpi_and_modules + nfc_module_height"
equation "\"enclosure_total_width\" = 2 * tolerances + 2 * wall_thickness + rpi_screen_width"
equation "\"enclosure_thickness\" = 40"
equation "\"enclosure_back_and_plate_distance\" = 3"
equation "\"enclosure_back_plate_thickness\" = 1.5"
equation "\"rpi_screen_screw_hole_diameter\" = 3"
equation "\"rpi_screen_top_screw_hole_side_distance\" = 2.5"
equation "\"rpi_screen_screw_post_depth\" = 13.6"
equation "\"rpi_screen_screw_post_diameter\" = 5.5"
equation "\"rpi_screen_screw_resting_plate_thickness\" = 2.7"
equation "\"nfc_module_standoff_inner_diameter\" = 4.5"
equation "\"rpi_camera_standoff_inner_diameter\" = 3.2"
equation "\"nfc_module_standoff_thickness\" = 2"
equation "\"rpi_camera_standoff_thickness\" = 3"
equation "\"nfc_module_standoff_depth\" = 3"
equation "\"rpi_camera_standoff_depth\" = 2.5"
equation "\"rpi_camera_screw_hole_vertical_apart\" = 12"
equation "\"rpi_camera_screw_hole_horizontal_apart\" = 20.2"
equation "\"rpi_camera_bottom_right_placement\" = 10"
equation "\"rpi_camera_hole_diameter\" = 13"
equation "\"suction_cup_distance_from_base\" = 25"
equation "\"suction_cup_inner_diameter\" = 13.5"
equation "\"suction_cup_nub_diameter\" = 14.5"
equation "\"suction_cup_inner_depth\" = 2.4"
equation "\"suction_cup_nub_depth\" = 3.8"
equation "\"usb_c_cutout_left_wall_distance\" = 21"
equation "\"usb_c_cutout_screen_distance\" = 15.5"
equation "\"usb_c_cutout_width\" = 15.5"
equation "\"back_plate_standoff_inner_diameter\" = 4.5"
equation "\"back_plate_standoff_thickness\" = 2"
equation "\"back_plate_standoff_screw_length\" = 8"
equation "\"back_plate_standoff_depth\" = 32"
equation "\"back_plate_standoff_heat_set_insert_depth\" = 3"
equation "\"back_plate_standoff_from_bottom\" = 2"
equation "\"rpi_screen_top_bottom_screw_hole_separation\" = 67.4"
equation "\"rpi_camera_standoff_depth_offset\" = 6.5"
equation "\"user_touch_edge_fillets\" = 2"
equation "\"suction_cup_arm_fillets\" = 5"
equation "\"rpi_screen_top_screw_hole_offset\" = 2.1"
equation "\"rpi_screen_bottom_screw_hole_anchor_length\" = 2.85"
equation "\"fan_length\" = 41"
equation "\"fan_depth\" = 11"
